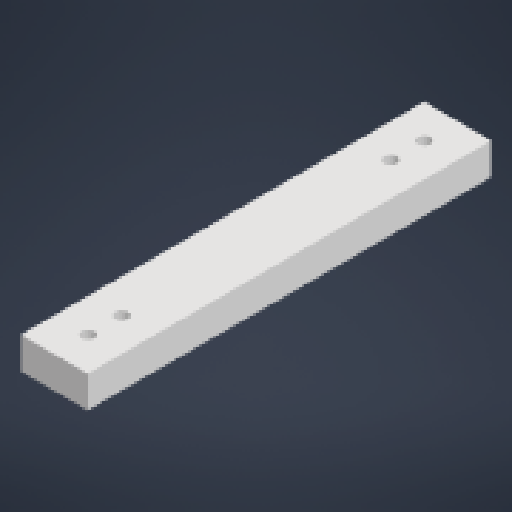
# Autodesk Inventor part: linkage
Saved by Autodesk Inventor 2023 (Build 270158000, 158)
## iProperties
Created: 2023-01-24
Part Number: linkage
Material: Generic
Document SubType Name: Modeling
Designer: Blank Slate
Density: 1 g/cm^3
Appearance: Default
Author: Blank Slate
Autodesk Inventor part; units mm, degrees
ref_plane "YZ Plane" through (0, 0, 0) normal (1, 0, 0) x (0, 1, 0)
ref_plane "XZ Plane" through (0, 0, 0) normal (0, 1, 0) x (-1, 0, 0)
ref_plane "XY Plane" through (0, 0, 0) normal (0, 0, 1) x (1, 0, 0)
sketch "Sketch1" plane through (0, 0, 0) normal (0, 1, 0) x (-1, 0, 0)
  line L0 (-344.259, 244.73) -> (-369.659, 244.73)
  line L1 (-369.659, 244.73) -> (-369.659, 92.33)
  line L2 (-369.659, 92.33) -> (-344.259, 92.33)
  line L3 (-344.259, 92.33) -> (-344.259, 244.73)
  line L4 (-356.959, 244.73) -> (-356.959, 219.33)
  line L5 (-356.959, 92.33) -> (-356.959, 117.73)
  line L6 (-356.959, 92.33) -> (-331.559, 92.33) construction
  circle A0 centre (-356.959, 219.33) radius 2.3813
  circle A1 centre (-356.959, 117.73) radius 2.3812
  circle A2 centre (-356.959, 232.03) radius 2.3813
  circle A3 centre (-356.959, 105.03) radius 2.3812
  point P0 (0, 0)
  dimension "d0" = 25.4
  dimension "d1" = 152.4
  dimension "d2" = 25.4
  dimension "d3" = 25.4
  dimension "d4" = 90
  dimension "d5" = 4.7625
  dimension "d6" = 4.7625
  dimension "d7" = 4.7625
  dimension "d8" = 4.7625
  constraints: 14 end point, 4 centre point, 4 midpoint, 2 coincident, 2 horizontal, 2 parallel, 2 perpendicular, 2 vertical
  measures "d0" distance of L2.end L1.end
  measures "d1" distance of L1.end L0.end
  measures "d2" distance of L4.start L4.end
  measures "d3" distance of L5.start L5.end
  measures "d4" angle of L6 L5
  measures "d5" diameter of A0
  measures "d6" diameter of A1
  measures "d7" diameter of A2
  measures "d8" diameter of A3
extrude "Extrusion1" add sketch "Sketch1" along normal blind 11.938
body "Solid1"
